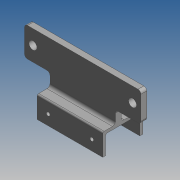
# Autodesk Inventor part: P047_BoitierCouvercleV4_porteLidar
Saved by Autodesk Inventor 2021.3 (Build 253353000, 353)
## iProperties
Created: 2022-01-14
Part Number: P047_BoitierCouvercleV4_porteLidar
Material: Générique
Document SubType Name: Modeling
Designer: gabri
Density: 1 g/cm^3
Appearance: Par défaut
Author: gabri
Autodesk Inventor part; units mm, degrees
ref_plane "YZ Plane" through (0, 0, 0) normal (1, 0, 0) x (0, 1, 0)
ref_plane "XZ Plane" through (0, 0, 0) normal (0, 1, 0) x (-1, 0, 0)
ref_plane "XY Plane" through (0, 0, 0) normal (0, 0, 1) x (1, 0, 0)
sketch "Sketch2" plane through (0, 0, 0) normal (0, 1, 0) x (-1, 0, 0)
  line L0 (22.5, -20) -> (-22.5, -20)
  line L1 (-22.5, -20) -> (-22.5, -30.9)
  line L2 (-22.5, -30.9) -> (22.5, -30.9)
  line L3 (22.5, -30.9) -> (22.5, -20)
  line L4 (0, -37.08) -> (0, 6.18) construction
  line L5 (40, 0) -> (-40, 0)
  line L6 (-40, 0) -> (-40, -20)
  line L7 (-40, -20) -> (40, -20)
  line L8 (40, -20) -> (40, 0)
  circle A0 centre (34.25, -10) radius 2.75
  circle A1 centre (-34.25, -10) radius 2.75
  point P0 (0, 0)
  point P1 (0, -20)
  point P2 (-22.5, -20)
  dimension "d0" = 45
  dimension "d1" = 22.5
  dimension "d2" = 10.9
  dimension "d3" = 5.5
  dimension "d4" = 68.5
  dimension "d5" = 34.25
  dimension "d6" = 40
  dimension "d7" = 40
  dimension "d8" = 20
  dimension "d9" = 10
  dimension "d10" = 5.5
  dimension "d11" = 10
  constraints: 16 end point, 4 parallel, 3 midpoint, 2 centre point, 2 horizontal, 2 perpendicular
  measures "d0" distance between parallel lines of L1 L3
  measures "d1" distance between parallel lines of L4 L3
  measures "d2" distance of L0.end L1.end
  measures "d3" diameter of A0
  measures "d4" distance of A1.centre A0.centre
  measures "d5" distance from line of L4 A0.centre
  measures "d6" distance between parallel lines of L4 L8
  measures "d7" distance between parallel lines of L6 L4
  measures "d8" distance between parallel lines of L5 L7
  measures "d9" distance from line of L5 A0.centre
  measures "d10" diameter of A1
  measures "d11" distance from line of L5 A1.centre
extrude "Extrusion1" add sketch "Sketch2" along normal blind 4
sketch "Sketch3" plane through (22.5, 0, -20) normal (1, 0, 0) x (0, 0, -1)
  line L0 (0, 0) -> (10.9, 0) construction
  line L1 (10.9, 0) -> (10.9, 4) construction
  line L2 (0, 4) -> (10.9, 4) construction
  line L3 (0, 0) -> (0, 4) construction
  line L4 (10.9, 4) -> (8.9, 4)
  line L5 (8.9, 4) -> (8.9, 17.75)
  line L6 (9.9, 18.75) -> (10.9, 18.75)
  line L7 (10.9, 15.75) -> (10.9, 4)
  line L8 (10.9, 18.75) -> (23.9, 18.75)
  line L9 (23.9, 18.75) -> (23.9, 16.75)
  line L10 (23.9, 16.75) -> (11.9, 16.75)
  line L11 (8.9, 0) -> (10.9, 0)
  line L12 (10.9, 0) -> (10.9, -5.75)
  line L13 (10.9, -8.75) -> (9.9, -8.75)
  line L14 (8.9, -7.75) -> (8.9, 0)
  line L15 (10.9, -8.75) -> (23.9, -8.75)
  line L16 (23.9, -8.75) -> (23.9, -6.75)
  line L17 (23.9, -6.75) -> (11.9, -6.75)
  arc A0 (11.9, 16.75) -> (10.9, 15.75) centre (11.9, 15.75) ccw
  arc A1 (9.9, 18.75) -> (8.9, 17.75) centre (9.9, 17.75) ccw
  arc A2 (8.9, -7.75) -> (9.9, -8.75) centre (9.9, -7.75) ccw
  arc A3 (10.9, -5.75) -> (11.9, -6.75) centre (11.9, -5.75) ccw
  point P0 (-20, 0)
  dimension "d14" = 6.75
  dimension "d15" = 12.75
  dimension "d16" = 2
  dimension "d17" = 2
  dimension "d18" = 2
  dimension "d19" = 13
  dimension "d20" = 1
  dimension "d21" = 15
  constraints: 28 end point, 8 point on circle, 8 tangent, 6 parallel, 5 point on line, 4 centre point, 4 horizontal, 4 perpendicular, 3 equal radius
  measures "d14" distance between parallel lines of L17 L11
  measures "d15" distance between parallel lines of L2 L10
  measures "d16" distance between parallel lines of L10 L8
  measures "d17" distance between parallel lines of L7 L5
  measures "d18" distance between parallel lines of L17 L15
  measures "d19" distance between parallel lines of L16 L12
  measures "d20" radius of A0
  measures "d21" distance between parallel lines of L5 L9
extrude "Extrusion2" add sketch "Sketch3" against normal up to surface (45 mm away)
fillet "Fillet1" radius 2 2 edges at (0, 0, -28.9) (0, 4, -28.9)
sketch "Sketch4" plane through (22.5, 18.75, -29.9) normal (0, 1, 0) x (1, 0, 0)
  line L0 (-45, 14) -> (-45, 0) construction
  line L1 (0, 0) -> (-45, 0) construction
  line L2 (0, 14) -> (0, 0) construction
  line L3 (0, 14) -> (-45, 14) construction
  line L4 (-22.5, 26.78) -> (-22.5, -62.68) construction
  point P0 (-22.5, -29.9)
  point P1 (-37.5, 7)
  point P2 (-7.5, 7)
  dimension "d25" = 15
  dimension "d26" = 15
  dimension "d27" = 7
  dimension "d28" = 7
  measures "d25" distance from line of L4 point (-37.5, 7)
  measures "d26" distance from line of point (-7.5, 7) L4
  measures "d27" distance from line of L3 point (-37.5, 7)
  measures "d28" distance from line of L3 point (-7.5, 7)
hole "Hole1" at (15, 18.75, -36.9) at (-15, 18.75, -36.9) direction (0, -1, 0) diameter 2.459 depth 27.5 thread size "M3x0.5" class "6H" standard "ISO Metric profile"
fillet "Fillet2" radius 2 6 edges at (22.5, 2, -20) (40, 2, -20) (40, 2, 0) (-40, 2, 0) (-40, 2, -20) (-22.5, 2, -20)
equation "\"d5\" = 0.5 * d4"
equation "\"d9\" = 0.5 * d8"
body "Solid1"
